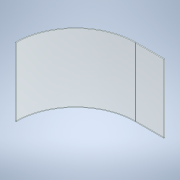
# Autodesk Inventor part: External Lexan
Saved by Autodesk Inventor 2020 (Build 240168000, 168)
## iProperties
Created: 2021-01-17
Part Number: External Lexan
Material: Glass
Document SubType Name: Modeling
Designer: magda
Density: 2.18 g/cm^3
Appearance: Clear
Author: magda
Autodesk Inventor part; units mm, degrees
ref_plane "YZ Plane" through (0, 0, 0) normal (1, 0, 0) x (0, 1, 0)
ref_plane "XZ Plane" through (0, 0, 0) normal (0, 1, 0) x (-1, 0, 0)
ref_plane "XY Plane" through (0, 0, 0) normal (0, 0, 1) x (1, 0, 0)
sketch "Sketch1" plane through (0, 0, 0) normal (0, 1, 0) x (-1, 0, 0)
  circle A0 centre (0, 0) radius 209.55
  circle A1 centre (0, 0) radius 212.725
  line L0 (0, 0) -> (246.9805, 0)
  line L1 (246.9805, 0) -> (246.9805, -270.6457)
  line L2 (246.9805, -270.6457) -> (0, -270.6457)
  line L3 (0, -270.6457) -> (0, 0)
  point P0 (0, -209.55)
  point P1 (0, -212.725)
  point P2 (212.725, 0)
  point P3 (209.55, 0)
  dimension "d0" = 419.1
  dimension "d1" = 425.45
  constraints: 8 end point, 2 centre point, 2 coincident, 2 parallel, 1 horizontal, 1 perpendicular
  measures "d0" diameter of A0
  measures "d1" diameter of A1
extrude "Extrusion1" add sketch "Sketch1" along normal blind 241.3 contours L0 A1 L3 A0 picked at (211.3642, -6.5426)
sketch "Sketch2" plane through (0, 0, -212.725) normal (1, 0, 0) x (0, 0, -1)
  line L0 (0, 0) -> (-212.725, 0) projected
  line L1 (0, 241.3) -> (-212.725, 241.3) projected
  line L2 (0, 0) -> (-3.1687, 0)
  line L3 (-3.1687, 0) -> (-3.1687, 241.3)
  line L4 (-3.1687, 241.3) -> (0, 241.3)
  line L5 (0, 241.3) -> (0, 0)
  point P0 (-3.1687, 0)
  constraints: 8 end point, 2 parallel, 1 horizontal, 1 perpendicular, 1 point on line
extrude "Extrusion2" add sketch "Sketch2" along normal blind 101.6
body "Solid1"
